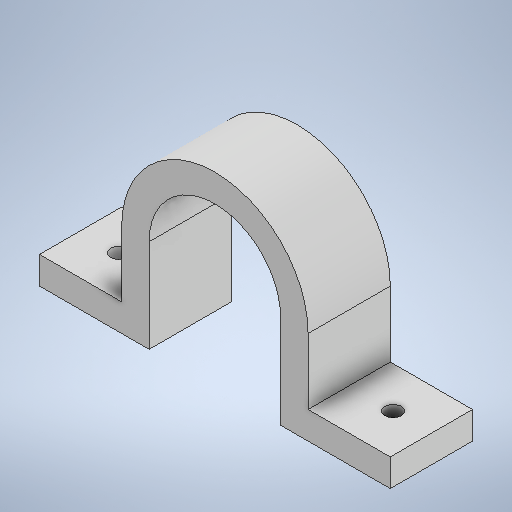
# Autodesk Inventor part: U_BRACKET_2
Saved by Autodesk Inventor 2025.3 (Build 293356030, 356C)
## iProperties
Created: 2026-06-30
Part Number: U_BRACKET_2
Material: Generic
Document SubType Name: Modeling
Designer: user
Density: 1 g/cm^3
Appearance: Default
Author: user
Autodesk Inventor part; units mm, degrees
ref_plane "YZ Plane" through (0, 0, 0) normal (1, 0, 0) x (0, 1, 0)
ref_plane "XZ Plane" through (0, 0, 0) normal (0, 1, 0) x (-1, 0, 0)
ref_plane "XY Plane" through (0, 0, 0) normal (0, 0, 1) x (1, 0, 0)
sketch "Sketch1" plane through (0, 0, 0) normal (0, 0, 1) x (1, 0, 0)
  line L0 (64, 0) -> (64, 5)
  line L1 (0, 5) -> (0, 0)
  arc A0 (49, 17) -> (15, 17) centre (32, 17) ccw
  line L2 (15, 5) -> (15, 17)
  line L3 (49, 5) -> (49, 17)
  line L4 (20, 0) -> (20, 17)
  arc A1 (44, 17) -> (20, 17) centre (32, 17) ccw
  line L5 (44, 17) -> (44, 0)
  line L6 (64, 5) -> (49, 5)
  line L7 (15, 5) -> (0, 5)
  line L8 (0, 0) -> (20, 0)
  line L9 (44, 0) -> (64, 0)
  dimension "d1" = 5
  dimension "d3" = 17
  dimension "d4" = 15
  dimension "d6" = 5
  dimension "d7" = 15
  dimension "d8" = 20
  constraints: 20 end point, 5 parallel, 4 point on circle, 2 centre point, 2 horizontal, 2 perpendicular, 2 tangent, 2 vertical
  measures "d1" distance of L0.end L0.start
  measures "d3" radius of A0
  measures "d4" distance between parallel lines of L1 L2
  measures "d6" radial gap between concentric circles of A0 A1
  measures "d7" distance from line of L3.start L0
  measures "d8" distance of L5.end L0.start
extrude "Extrusion1" add sketch "Sketch1" along normal blind 15
sketch "Sketch2" plane through (0, 5, 0) normal (0, 1, 0) x (1, 0, 0)
  line L0 (15, 0) -> (0, 0) projected
  line L1 (64, 0) -> (49, 0) projected
  line L2 (0, 0) -> (0, -15) projected
  point P0 (7, -7.5)
  point P1 (57, -7.5)
  dimension "d18" = 50
  dimension "d19" = 7.5
  dimension "d20" = 7.5
  dimension "d21" = 7
  measures "d18" distance of point (57, -7.5) point (7, -7.5)
  measures "d19" distance from line of L0 point (7, -7.5)
  measures "d20" distance from line of L1 point (57, -7.5)
  measures "d21" distance from line of L2 point (7, -7.5)
hole "Hole1" at (7, 5, 7.5) at (57, 5, 7.5) direction (0, -1, 0) diameter 3 end through all
body "Solid1"
